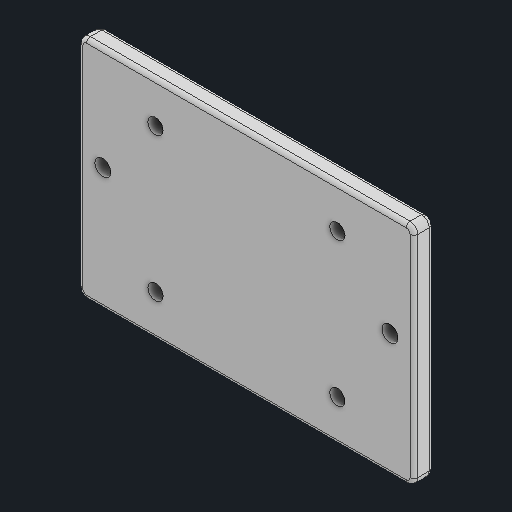
# Autodesk Inventor part: CylinderSupport
Saved by Autodesk Inventor 2025 (Build 290162000, 162)
## iProperties
Created: 2024-05-26
Part Number: CylinderSupport
Material: Generic
Document SubType Name: Modeling
Designer: zulet
Density: 1 g/cm^3
Appearance: Default
Author: zulet
Autodesk Inventor part; units mm, degrees
ref_plane "YZ Plane" through (0, 0, 0) normal (1, 0, 0) x (0, 1, 0)
ref_plane "XZ Plane" through (0, 0, 0) normal (0, 1, 0) x (-1, 0, 0)
ref_plane "XY Plane" through (0, 0, 0) normal (0, 0, 1) x (1, 0, 0)
sketch "Sketch1" plane through (0, 0, 0) normal (0, 0, 1) x (1, 0, 0)
  circle A0 centre (75, 150.5) radius 4.1881 projected
  circle A1 centre (75, 61.5) radius 4.1881 projected
  circle A2 centre (-75, 61.5) radius 4.1881 projected
  circle A3 centre (-75, 150.5) radius 4.1881 projected
  line L0 (-87.5, -2.5) -> (87.5, -2.5)
  line L1 (87.5, -2.5) -> (87.5, 115.5)
  line L2 (87.5, 115.5) -> (-87.5, 115.5)
  line L3 (-87.5, 115.5) -> (-87.5, -2.5)
  line L4 (-87.5, -2.5) -> (87.5, 115.5) construction
  line L5 (87.5, -2.5) -> (-87.5, 115.5) construction
  line L6 (47.5, 94) -> (-47.5, 94) construction
  line L7 (-47.5, 94) -> (-47.5, 19) construction
  line L8 (-47.5, 19) -> (47.5, 19) construction
  line L9 (47.5, 19) -> (47.5, 94) construction
  line L10 (47.5, 94) -> (-47.5, 19) construction
  line L11 (-47.5, 94) -> (47.5, 19) construction
  line L12 (75, 61.5) -> (-75, 61.5) construction
  line L13 (0, 61.5) -> (0, 56.5) construction
  point P0 (0, 0)
  dimension "d0" = 175
  dimension "d1" = 118
  dimension "d2" = 95
  dimension "d3" = 75
  dimension "d15" = 5
  constraints: 28 end point, 5 midpoint, 4 coincident, 4 parallel, 3 horizontal, 2 perpendicular, 1 vertical
  measures "d0" distance of L2.end L1.end
  measures "d1" distance of L1.end L0.end
  measures "d2" distance of L8.end L7.end
  measures "d3" distance of L7.end L6.end
  measures "d15" distance of L13.start L13.end
extrude "Extrusion1" add sketch "Sketch1" along normal blind 10 contours L3 L2 L1 L0
hole "Hole1" at (47.5, 94, 0) at (47.5, 19, 0) at (-47.5, 19, 0) at (-47.5, 94, 0) direction (0, 0, 1) diameter 8 depth 15
fillet "Fillet1" radius 4 4 edges at (87.5, 115.5, 5) (87.5, -2.5, 5) (-87.5, -2.5, 5) (-87.5, 115.5, 5)
fillet "Fillet2" radius 2 16 edges at (86.3284, 114.3284, 0) (0, 115.5, 0) (-86.3284, 114.3284, 0) (-87.5, 56.5, 0) (-86.3284, -1.3284, 0) (0, -2.5, 0) (86.3284, -1.3284, 0) (87.5, 56.5, 0) (86.3284, 114.3284, 10) (0, 115.5, 10) (-86.3284, 114.3284, 10) (-87.5, 56.5, 10) (-86.3284, -1.3284, 10) (0, -2.5, 10) (86.3284, -1.3284, 10) (87.5, 56.5, 10)
body "Solid1"
